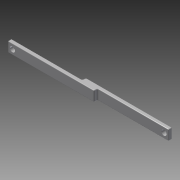
# Autodesk Inventor part: Diagonal Supporter
Saved by Autodesk Inventor 2013 (Build 170138000, 138)
## iProperties
Created: 2014-05-22
Part Number: Diagonal Supporter
Material: Steel
Document SubType Name: Modeling
Designer: nojessen
Mass: 740.348 g
Surface Area: 274.37 cm^2
Volume: 94.3118 cm^3
Density: 7.85 g/cm^3
Author: nojessen
Autodesk Inventor part; units mm, degrees
ref_plane "YZ Plane" through (0, 0, 0) normal (1, 0, 0) x (0, 1, 0)
ref_plane "XZ Plane" through (0, 0, 0) normal (0, 1, 0) x (-1, 0, 0)
ref_plane "XY Plane" through (0, 0, 0) normal (0, 0, 1) x (1, 0, 0)
sketch "Sketch1" plane through (0, 0, 0) normal (0, 0, 1) x (1, 0, 0)
  line L0 (0, 0) -> (393.7, 0)
  line L1 (393.7, 0) -> (393.7, 25.4)
  line L2 (393.7, 25.4) -> (0, 25.4)
  line L3 (0, 25.4) -> (0, 0)
  line L4 (0, 12.7) -> (11.43, 12.7) construction
  line L5 (393.7, 12.7) -> (382.27, 12.7) construction
  circle A0 centre (11.43, 12.7) radius 6.35
  circle A1 centre (382.27, 12.7) radius 6.35
  dimension "d0" = 393.7
  dimension "d1" = 25.4
  dimension "d2" = 11.43
  dimension "d3" = 11.43
  dimension "d4" = 12.7
  dimension "d5" = 12.7
  constraints: 12 end point, 3 equal length, 2 centre point, 2 coincident, 2 midpoint, 2 perpendicular, 1 horizontal
  measures "d0" distance of L2.end L1.end
  measures "d1" distance of L1.end L0.end
  measures "d2" distance of L4.start L4.end
  measures "d3" distance of L5.start L5.end
  measures "d4" diameter of A0
  measures "d5" diameter of A1
extrude "Extrusion1" add sketch "Sketch1" along normal blind 17.78
sketch "Sketch2" plane through (0, 25.4, 0) normal (0, 1, 0) x (1, 0, 0)
  line L0 (0, 0) -> (177.8069, 0)
  line L1 (177.8069, 0) -> (177.8069, -8.89)
  line L2 (177.8069, -8.89) -> (0, -8.89)
  line L3 (0, -8.89) -> (0, 0)
  line L4 (393.7, -17.78) -> (215.9, -17.78)
  line L5 (215.9, -17.78) -> (215.9, -8.89)
  line L6 (215.9, -8.89) -> (393.7, -8.89)
  line L7 (393.7, -8.89) -> (393.7, -17.78)
  dimension "d8" = 177.8
  constraints: 16 end point, 4 parallel, 2 horizontal, 2 perpendicular
  measures "d8" distance of L5.end L6.end
extrude "Extrusion2" cut sketch "Sketch2" against normal blind 50.8
fillet "Fillet1" radius 3.175 4 edges at (215.9, 12.7, 8.89) (215.9, 12.7, 17.78) (177.8069, 12.7, 8.89) (177.8069, 12.7, 0)
fillet "Fillet2" radius 1.5875 28 edges at (178.7368, 25.4, 0.9299) (177.8069, 25.4, 4.445) (176.877, 25.4, 7.9601) (87.3159, 25.4, 8.89) (287.3409, 25.4, 0) (216.8299, 25.4, 9.8199) (215.9, 25.4, 13.335) (214.9701, 25.4, 16.8501) (106.3625, 25.4, 17.78) (306.3875, 25.4, 8.89) (393.7, 25.4, 4.445) (393.7, 12.7, 8.89) (393.7, 12.7, 0) (178.7368, 0, 0.9299) (177.8069, 0, 4.445) (176.877, 0, 7.9601) (87.3159, 0, 8.89) (287.3409, 0, 0) (393.7, 0, 4.445) (216.8299, 0, 9.8199) (215.9, 0, 13.335) (214.9701, 0, 16.8501) (106.3625, 0, 17.78) (306.3875, 0, 8.89) (0, 12.7, 17.78) (0, 25.4, 13.335) (0, 12.7, 8.89) (0, 0, 13.335)
fillet "Fillet3" radius 0.3175 4 edges at (5.08, 12.7, 17.78) (5.08, 12.7, 8.89) (375.92, 12.7, 0) (375.92, 12.7, 8.89)
body "Solid1"
